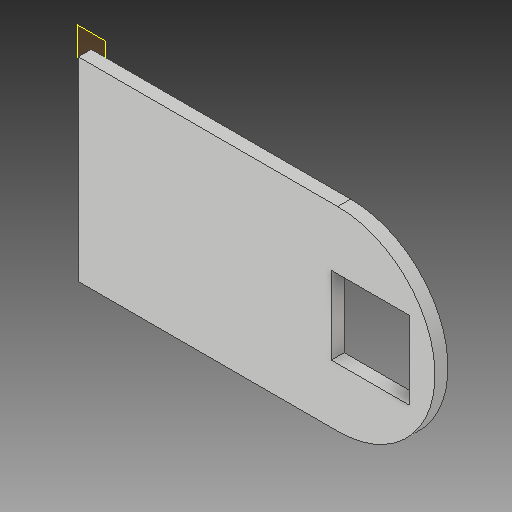
# Autodesk Inventor part: Основание
Saved by Autodesk Inventor 2018.3 (Build 223284000, 284)
## iProperties
Created: 1900-01-01
Part Number: Основание
Material: Типовые
Document SubType Name: Modeling
Designer: Leancher
Density: 1 g/cm^3
Appearance: По умолчанию
Author: Leancher
Revision Number: ANYUNSPECIFIED
Autodesk Inventor part; units mm, degrees
ref_plane "YZ Plane" through (0, 0, 0) normal (1, 0, 0) x (0, 1, 0)
ref_plane "XZ Plane" through (0, 0, 0) normal (0, 1, 0) x (-1, 0, 0)
ref_plane "XY Plane" through (0, 0, 0) normal (0, 0, 1) x (1, 0, 0)
ref_plane "РабПлоскость1" through (-120, 75, 10) normal (0, 0, 1) x (1, 0, 0)
sketch "Эскиз1" plane through (-120, 75, 10) normal (0, 0, 1) x (1, 0, 0)
  line L0 (199.9778, 0) -> (0, 0)
  line L1 (0, 0) -> (0, -150)
  line L2 (0, -150) -> (199.9778, -150)
  arc A0 (199.9778, -150) -> (199.9778, 0) centre (199.9778, -75) ccw
  line L3 (194.9778, -45) -> (194.9778, -105)
  line L4 (194.9778, -105) -> (254.9778, -105)
  line L5 (254.9778, -105) -> (254.9778, -45)
  line L6 (194.9778, -45) -> (254.9778, -45)
  dimension "d4" = 60
  dimension "d5" = 60
  constraints: 14 end point, 2 perpendicular, 2 point on circle, 1 centre point, 1 horizontal
  measures "d4" distance of L3.start L3.end
  measures "d5" distance of L3.end L4.end
extrude "Выдавливание1" add sketch "Эскиз1" along normal blind 10
